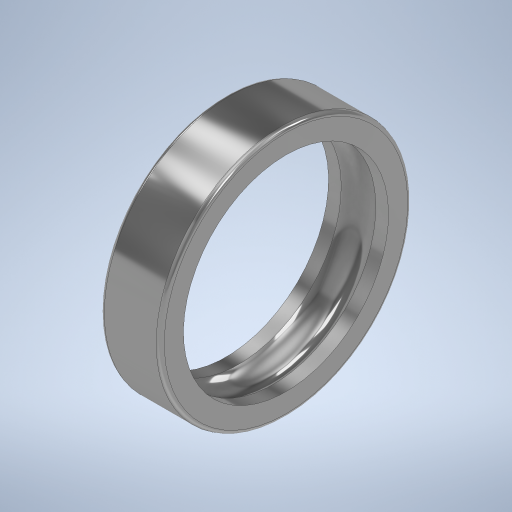
# Autodesk Inventor part: Outer Ring(fixed)
Saved by Autodesk Inventor 2023 (Build 270158000, 158)
## iProperties
Created: 2023-03-23
Part Number: Outer Ring(fixed)
Material: Generic
Document SubType Name: Modeling
Designer: CASPER
Density: 1 g/cm^3
Appearance: Chrome - Polished Black
Author: CASPER
Autodesk Inventor part; units mm, degrees
ref_plane "YZ Plane" through (0, 0, 0) normal (1, 0, 0) x (0, 1, 0)
ref_plane "XZ Plane" through (0, 0, 0) normal (0, 1, 0) x (-1, 0, 0)
ref_plane "XY Plane" through (0, 0, 0) normal (0, 0, 1) x (1, 0, 0)
sketch "Sketch2" plane through (0, 0, 0) normal (0, 0, 1) x (1, 0, 0)
  line L0 (1.55, 6.5) -> (-1.55, 6.5)
  line L1 (-1.55, 6.5) -> (-1.55, 5.3)
  line L2 (-1.55, 5.3) -> (1.55, 5.3)
  line L3 (1.55, 5.3) -> (1.55, 6.5)
  arc A0 (0.8944, 5.3) -> (-0.8944, 5.3) centre (0, 4.5) ccw
  line L4 (-2.17, 0) -> (2.17, 0) projected
  point P0 (0, 0)
  dimension "d8" = 3.1
  dimension "d9" = 1.2
  dimension "d10" = 1.55
  dimension "d11" = 5.3
  dimension "d12" = 0.8
  dimension "d13" = 1.2
  constraints: 8 end point, 2 parallel, 2 point on circle, 2 point on line, 1 centre point, 1 horizontal, 1 perpendicular, 1 vertical alignment
  measures "d8" distance of L0.start L0.end
  measures "d9" distance of L0.end L1.end
  measures "d10" horizontal distance of point (0, 0) L1.end
  measures "d11" vertical distance of point (0, 0) L2.end
  measures "d12" distance from line of L2 A0.centre
  measures "d13" radius of A0
revolve "Revolution2" add sketch "Sketch2" angle 360 about axis through (-10, 0, 0) along (1, 0, 0) contours L3 L2 A0 L1 L0
fillet "Fillet1" radius 0.21 2 edges at (1.55, -6.5, 0) (-1.55, -6.5, 0)
body "Solid2"
